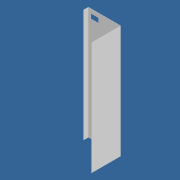
# Autodesk Inventor part: Controller_Panel
Saved by Autodesk Inventor 2020 (Build 240168000, 168)
## iProperties
Created: 2021-05-17
Part Number: Controller_Panel
Material: 一般
Document SubType Name: Sheet Metal
Designer: ken113
Density: 1 g/cm^3
Sheet Metal Rule: Default_mm
Appearance: 既定
Author: ken113
Autodesk Inventor part; units mm, degrees
ref_plane "YZ Plane" through (0, 0, 0) normal (1, 0, 0) x (0, 1, 0)
ref_plane "XZ Plane" through (0, 0, 0) normal (0, 1, 0) x (-1, 0, 0)
ref_plane "XY Plane" through (0, 0, 0) normal (0, 0, 1) x (1, 0, 0)
sketch "スケッチ1" plane through (0, 0, 0) normal (0, 0, 1) x (1, 0, 0)
  line L0 (100, -345) -> (-100, -345)
  line L1 (-100, -345) -> (-100, 345)
  line L2 (-100, 345) -> (100, 345)
  line L3 (100, 345) -> (100, -345)
  line L4 (100, -345) -> (-100, 345) construction
  line L5 (-100, -345) -> (100, 345) construction
  point P0 (0, 0)
  dimension "d0" = 200
  dimension "d1" = 690
  measures "d0" distance of L1.end L2.end
  measures "d1" distance of L0.end L1.end
extrude "プレート1" add sketch "スケッチ1" along normal blind 1.5
sketch "スケッチ2" plane through (-98.5, -345, 0) normal (-1, 0, 0) x (0, -1, 0)
  line L0 (-690, 0) -> (0, 0)
  line L1 (0, 0) -> (0, 30)
  line L2 (0, 30) -> (-690, 30)
  line L3 (-690, 30) -> (-690, 0)
  constraints: 6 end point, 1 horizontal, 1 perpendicular, 1 vertical
edge flange "フランジ1" height 30 angle 90 thickness 1.5 bend radius 1.5 thickness toward (-1, 0, 0) relief straight relief width 1.5 relief depth 0.75 edges at (-100, 0, 1.5) wall of the first edge with corners at (-98.5, 345, 0) (-98.5, -345, 0) (-98.5, -345, 30) (-98.5, 345, 30)
bend "曲げ1"
corner "コーナー1"
sketch "スケッチ6" plane through (0, 0, 0) normal (0, 0, -1) x (-1, 0, 0)
  line L0 (36.5, 291) -> (83.5, 291)
  line L1 (83.5, 291) -> (83.5, 319)
  line L2 (83.5, 319) -> (36.5, 319)
  line L3 (36.5, 319) -> (36.5, 291)
  line L4 (36.5, 291) -> (83.5, 319) construction
  line L5 (83.5, 291) -> (36.5, 319) construction
  line L6 (97, 345) -> (-100, 345) projected
  line L7 (100, 345) -> (100, -345) projected
  point P0 (0, 0)
  point P1 (60, 305)
  dimension "d40" = 47
  dimension "d41" = 28
  dimension "d83" = 40
  dimension "d84" = 40
  constraints: 12 end point, 2 midpoint, 2 parallel, 1 horizontal, 1 perpendicular
  measures "d40" distance of L2.end L1.end
  measures "d41" distance of L1.end L0.end
  measures "d83" distance from line of L6 point (60, 305)
  measures "d84" distance from line of L7 point (60, 305)
extrude "押し出し2" cut sketch "スケッチ6" against normal blind 10
sketch "スケッチ7" plane through (0, 0, 0) normal (0, 0, -1) x (-1, 0, 0)
  line L0 (36.5, 291) -> (36.5, 319) projected
  line L1 (36.5, 319) -> (83.5, 319) projected
  line L2 (83.5, 319) -> (83.5, 291) projected
  line L3 (83.5, 291) -> (36.5, 291) projected
  line L4 (97, -345) -> (97, 345) projected
  line L5 (83.5, 319) -> (83.5, 291) projected
  line L6 (36.5, 319) -> (83.5, 319) projected
  line L7 (-100, -345) -> (97, -345) projected
  line L8 (97, 345) -> (-100, 345) projected
  line L9 (-100, 345) -> (-100, -345) projected
  line L10 (83.5, 291) -> (36.5, 291) projected
  point P0 (0, 0)
  point P1 (88, 305)
  point P2 (32, 305)
  point P3 (83.5, 305)
  point P4 (83.5, 305)
  point P5 (60, 291)
  dimension "d85" = 56
  dimension "d86" = 28
  constraints: 3 midpoint, 2 horizontal alignment
  measures "d85" distance of point (32, 305) point (88, 305)
  measures "d86" horizontal distance of point (32, 305) point (60, 291)
hole "穴2" at (-88, 305, 0) at (-32, 305, 0) direction (0, 0, 1) diameter 3.2 end through all
fillet "フィレット1" radius 2 4 edges at (-36.5, 291, 0.75) (-83.5, 291, 0.75) (-36.5, 319, 0.75) (-83.5, 319, 0.75)
sketch "スケッチ9" plane through (98.5, 345, 0) normal (1, 0, 0) x (0, 1, 0)
  line L0 (-690, 0) -> (0, 0)
  line L1 (0, 0) -> (0, 180)
  line L2 (0, 180) -> (-690, 180)
  line L3 (-690, 180) -> (-690, 0)
  constraints: 6 end point, 1 horizontal, 1 perpendicular, 1 vertical
edge flange "フランジ3" height 180 angle 90 thickness 1.5 bend radius 1.5 thickness toward (1, 0, 0) relief straight relief width 1.5 relief depth 0.75 edges at (100, 0, 1.5) wall of the first edge with corners at (98.5, -345, 0) (98.5, 345, 0) (98.5, 345, 180) (98.5, -345, 180)
bend "曲げ3"
corner "コーナー3"
equation "\"d53\" = Thickness"
equation "\"d2\" = Thickness"
equation "\"d3\" = BendReliefWidth"
equation "\"d4\" = BendReliefDepth"
equation "\"d5\" = MinimumRemnant"
equation "\"d6\" = TransitionRadius"
equation "\"d9\" = BendRadius"
equation "\"d10\" = CornerReliefSize"
equation "\"d11\" = GapSize"
equation "\"d12\" = JacobiRadiusSize"
equation "\"d73\" = BendReliefWidth"
equation "\"d74\" = BendReliefDepth"
equation "\"d75\" = MinimumRemnant"
equation "\"d76\" = TransitionRadius"
equation "\"d79\" = BendRadius"
equation "\"d80\" = CornerReliefSize"
equation "\"d81\" = GapSize"
equation "\"d82\" = JacobiRadiusSize"
equation "\"BendRadius\" = Thickness"
equation "\"BendReliefWidth\" = Thickness"
equation "\"BendReliefDepth\" = 0.5 * Thickness"
equation "\"CornerReliefSize\" = 4 * Thickness"
equation "\"MinimumRemnant\" = 2 * Thickness"
equation "\"TransitionRadius\" = BendRadius"
equation "\"JacobiRadiusSize\" = BendRadius"
equation "\"GapSize\" = Thickness"
equation "\"Thickness\" = 1.5"
